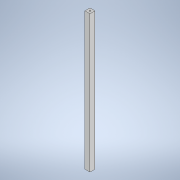
# Autodesk Inventor part: P_3030_1500
Saved by Autodesk Inventor 2020 (Build 240168000, 168)
## iProperties
Created: 2022-04-08
Part Number: P_3030_1500
Material: Genérico
Document SubType Name: Modeling
Designer: aarco
Density: 1 g/cm^3
Appearance: Valor por defecto
Author: aarco
Autodesk Inventor part; units mm, degrees
ref_plane "YZ Plane" through (0, 0, 0) normal (1, 0, 0) x (0, 1, 0)
ref_plane "XZ Plane" through (0, 0, 0) normal (0, 1, 0) x (-1, 0, 0)
ref_plane "XY Plane" through (0, 0, 0) normal (0, 0, 1) x (1, 0, 0)
sketch "Boceto1" plane through (0, 0, 0) normal (0, 1, 0) x (-1, 0, 0)
  line L0 (15, 15) -> (-15, 15)
  line L1 (-15, 15) -> (-15, -15)
  line L2 (-15, -15) -> (15, -15)
  line L3 (15, -15) -> (15, 15)
  line L4 (15, 15) -> (-15, -15) construction
  circle A0 centre (0, 0) radius 4
  dimension "d0" = 30
  dimension "d1" = 8
  constraints: 10 end point, 2 coincident, 2 parallel, 2 perpendicular, 1 centre point, 1 horizontal, 1 midpoint
  measures "d0" distance of L0.start L0.end
  measures "d1" diameter of A0
extrude "Extrusión1" add sketch "Boceto1" along normal blind 823
